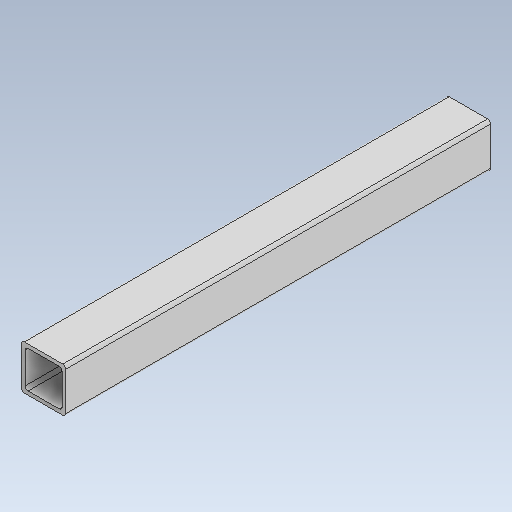
# Autodesk Inventor part: secure_width_bar
Saved by Autodesk Inventor 2021 (Build 250183000, 183)
## iProperties
Created: 2021-05-28
Part Number: secure_width_bar
Material: Generic
Document SubType Name: Modeling
Density: 1 g/cm^3
Appearance: Default
Autodesk Inventor part; units mm, degrees
ref_plane "YZ Plane" through (0, 0, 0) normal (1, 0, 0) x (0, 1, 0)
ref_plane "XZ Plane" through (0, 0, 0) normal (0, 1, 0) x (-1, 0, 0)
ref_plane "XY Plane" through (0, 0, 0) normal (0, 0, 1) x (1, 0, 0)
sketch "Sketch1" plane through (0, 0, 0) normal (1, 0, 0) x (0, 1, 0)
  line L0 (15, 143.75) -> (-15, 143.75)
  line L1 (-15, 143.75) -> (-15, -143.75)
  line L2 (-15, -143.75) -> (15, -143.75)
  line L3 (15, -143.75) -> (15, 143.75)
  point P0 (0, 0)
  dimension "d0" = 287.5
  dimension "d1" = 143.75
  dimension "d2" = 30
  dimension "d3" = 15
  constraints: 8 end point, 2 parallel, 1 horizontal, 1 perpendicular
  measures "d0" distance of L2.end L0.start
  measures "d1" distance from line of L0 point (0, 0)
  measures "d2" distance of L1.end L2.end
  measures "d3" distance from line of L3 point (0, 0)
extrude "Extrusion1" add sketch "Sketch1" along normal blind 30
fillet "Fillet1" radius 2 4 edges at (0, 15, 0) (0, -15, 0) (30, -15, 0) (30, 15, 0)
sketch "Sketch2" plane through (0, -13, -143.75) normal (0, 0, -1) x (-1, 0, 0)
  line L0 (-27.5, 25.5) -> (-2.5, 25.5)
  line L1 (-2.5, 25.5) -> (-2.5, 0.5)
  line L2 (-2.5, 0.5) -> (-27.5, 0.5)
  line L3 (-27.5, 0.5) -> (-27.5, 25.5)
  line L4 (-2, 28) -> (-28, 28) projected
  line L5 (-2, -2) -> (-28, -2) projected
  line L6 (0, 0) -> (0, 26) projected
  line L7 (-30, 0) -> (-30, 26) projected
  point P0 (0, 13)
  dimension "d7" = 2.5
  dimension "d8" = 2.5
  dimension "d9" = 2.5
  dimension "d10" = 2.5
  constraints: 8 end point, 2 parallel, 1 horizontal, 1 perpendicular
  measures "d7" distance between parallel lines of L4 L0
  measures "d8" distance between parallel lines of L5 L2
  measures "d9" distance between parallel lines of L6 L1
  measures "d10" distance between parallel lines of L7 L3
extrude "Extrusion2" cut sketch "Sketch2" against normal blind 300
fillet "Fillet2" radius 2 4 edges at (27.5, -12.5, 0) (27.5, 12.5, 0) (2.5, 12.5, 0) (2.5, -12.5, 0)
equation "\"d0\" = 0.5 * wheelchair_deployed_width - secure_arm_hold_thickness"
equation "\"d1\" = 0.5 * d0"
equation "\"d2\" = secure_arm_hold_thickness"
equation "\"d3\" = 0.5 * d2"
equation "\"d4\" = secure_arm_hold_thickness"
equation "\"hoop_angle_z\" = 45deg"
equation "\"hoop_bearing_length\" = 5deg"
equation "\"hoop_cable_diam\" = 5"
equation "\"hoop_cable_pulley_diam\" = 22"
equation "\"rack_tooth_addendum\" = 5"
equation "\"rack_tooth_dedendum\" = 5"
equation "\"rack_tooth_thickness\" = 5"
equation "\"secure_arm_angle\" = 35deg"
equation "\"secure_arm_hold_thickness\" = 30"
equation "\"secure_arm_radii\" = 9"
equation "\"support_baseClamp_platformLengthBuffer\" = 35"
equation "\"support_baseClamp_platformThickness\" = 15"
equation "\"support_baseClamp_platformWidthBuffer\" = 0"
equation "\"support_baseClamp_sleeveHoleDiameter\" = 12"
equation "\"support_baseClamp_sleeveSweepTerminationAngle\" = 55deg"
equation "\"support_baseClamp_thickness\" = 8"
equation "\"support_frame_endHoleBuffer\" = 25"
equation "\"support_frame_squareBarFillet\" = 2"
equation "\"support_frame_squareBarThickness\" = 5"
equation "\"hoop_tabs_thickness\" = 6"
equation "\"hoop_tabs_hole\" = 12"
equation "\"wheelchair_deployed_width\" = 635"
equation "\"wheelchair_deployed_height\" = 914"
equation "\"wheelchair_deployed_length\" = 1067"
equation "\"sm_varx_pinPlate_thickness\" = 5"
equation "\"sm_varx_member_tolerance\" = 0.5"
equation "\"sm_varx_pinPlate_holeDiameter\" = 5"
equation "\"sm_varx_squareBarThickness\" = 2.5"
body "Solid1"
